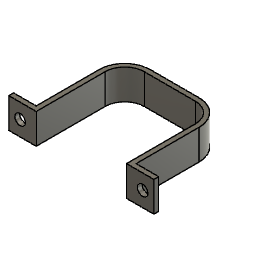
BatteryBracket (Autodesk Fusion 360 design; units mm, degrees)
Autodesk Fusion 360 part; units mm, degrees
sketch "Sketch1" plane through (0, 0, 0) normal (0, 1, 0) x (1, 0, 0)
  line L0 (0, 0) -> (-1.6, 0)
  line L1 (-1.6, 0) -> (-1.6, 31)
  line L2 (-1.6, 31) -> (0, 31)
  line L3 (0, 31) -> (0, 0)
  line L4 (7.5, 0) -> (0, 0)
  line L5 (0, 0) -> (0, 1.6)
  line L6 (0, 1.6) -> (7.5, 1.6)
  line L7 (7.5, 1.6) -> (7.5, 0)
  line L8 (-1.6, 31) -> (-31.6, 31)
  line L9 (-31.6, 31) -> (-31.6, 29.4)
  line L10 (-31.6, 29.4) -> (-1.6, 29.4)
  line L11 (-1.6, 29.4) -> (-1.6, 31)
  line L12 (-31.6, 31) -> (-33.2, 31)
  line L13 (-33.2, 31) -> (-33.2, 0)
  line L14 (-33.2, 0) -> (-31.6, 0)
  line L15 (-31.6, 0) -> (-31.6, 31)
  line L16 (-40.7, 1.6) -> (-33.2, 1.6)
  line L17 (-33.2, 1.6) -> (-33.2, 0)
  line L18 (-33.2, 0) -> (-40.7, 0)
  line L19 (-40.7, 0) -> (-40.7, 1.6)
  dimension "d2" = 1.6
  dimension "d3" = 7.5
  dimension "d4" = 1.6
  dimension "d5" = 1.6
  dimension "d6" = 1.6
  dimension "d7" = 30
  dimension "d16" = 29.4
  constraint horizontal L0
  constraint vertical L1
  constraint horizontal L2
  constraint vertical L3
  constraint coincident L0.start L3.end
  constraint horizontal L4
  constraint vertical L5
  constraint horizontal L6
  constraint vertical L7
  constraint coincident L3 L5.end
  constraint horizontal L8
  constraint vertical L9
  constraint horizontal L10
  constraint vertical L11
  constraint horizontal L12
  constraint vertical L13
  constraint horizontal L14
  constraint vertical L15
  constraint horizontal L16
  constraint vertical L17
  constraint horizontal L18
  constraint vertical L19
  constraint equal L1 L15
  constraint equal L6 L16
  constraint equal L7 L19
  measures "d2" distance of L1.end L2.end
  measures "d3" distance of L5.end L6.end
  measures "d4" distance of L4.start L6.end
  measures "d5" distance of L8 L10
  measures "d6" distance of L13 L15
  measures "d7" distance of L1.end L8.end
  measures "d16" distance of L0 L10
extrude "Extrude1" add sketch "Sketch1" along normal blind 10
hole "Hole1" at (3.75, 5, -1.6) direction (0, 0, 1) diameter 3.5 depth 4 tip angle 118
hole "Hole2" at (-36.95, 5, -1.6) direction (0, 0, 1) diameter 3.5 depth 4 tip angle 118
fillet "Fillet1" radius 6.5 2 edges at (-1.6, 5, -29.4) (-31.6, 5, -29.4)
fillet "Fillet2" radius 8.5 2 edges at (0, 5, -31) (-33.2, 5, -31)
equation "d2 = d4"
equation "d5 = d4"
equation "d6 = d4"
